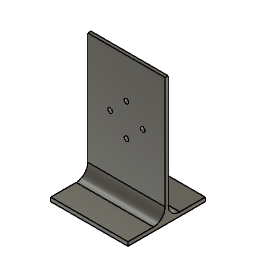
support-motor-v4 (Autodesk Fusion 360 design; units mm, degrees)
Autodesk Fusion 360 part; units mm, degrees
note: some values were not read from the file. Set by a fixed rule: which sketch regions a step uses.
sketch "Sketch1" plane through (0, 0, 0) normal (0, 0, 1) x (1, 0, 0)
  line L0 (0, 0) -> (50, 0)
  line L1 (50, 0) -> (50, 50)
  line L2 (50, 50) -> (0, 50)
  line L3 (0, 50) -> (0, 0)
  dimension "d3" = 50
  dimension "d4" = 50
  constraint horizontal L0
  constraint vertical L1
  constraint horizontal L2
  constraint vertical L3
  constraint coincident L0.start L3.end
  measures "d3" distance of L1.end L2.end
  measures "d4" distance of L0.start L2.end
extrude "Extrude1" add sketch "Sketch1" along normal blind 2.5
sketch "Sketch2" plane through (0, 0, 2.5) normal (0, 0, 1) x (-1, 0, 0)
  line L0 (0, -50) -> (0, 0)
  line L1 (0, 0) -> (-50, 0)
  line L2 (-50, 0) -> (-50, -50)
  line L3 (-50, -50) -> (0, -50)
  line L4 (0, -25) -> (-50, -25)
  line L5 (0, -26) -> (-50, -26)
  line L6 (-50, -26) -> (-50, -24)
  line L7 (-50, -24) -> (0, -24)
  line L8 (0, -24) -> (0, -26)
  dimension "d5" = 1
  dimension "d6" = 1
  constraint midpoint L0 L4.start
  constraint midpoint L2 L4.end
  constraint horizontal L5
  constraint vertical L6
  constraint horizontal L7
  constraint vertical L8
  constraint coincident L2 L6.end
  constraint coincident L0 L5.start
  measures "d5" distance of L4 L5
  measures "d6" distance of L4 L7
extrude "Extrude2" add sketch "Sketch2" along normal blind 80 contours L0 L2 L4 L5 L6 L8 | L0 L2 L4 L6 L7 L8
fillet "Fillet1" radius 7.5 2 edges at (25, 24, 2.5) (25, 26, 2.5)
sketch "Sketch3" plane through (0, 24, 0) normal (0, -1, 0) x (1, 0, 0)
  line L0 (0, 10) -> (50, 10)
  line L1 (50, 10) -> (50, 82.5)
  line L2 (50, 82.5) -> (0, 82.5)
  line L3 (0, 82.5) -> (0, 10)
  line L4 (0, 46.25) -> (50, 46.25)
  line L5 (25, 82.5) -> (25, 0)
  circle A0 centre (25, 56.75) radius 1.5
  circle A1 centre (14.5, 46.25) radius 1.5
  circle A2 centre (35.5, 46.25) radius 1.5
  circle A3 centre (25, 35.75) radius 1.5
  dimension "d11" = 3
  dimension "d12" = 10.5
  dimension "d13" = 3
  dimension "d14" = 10.5
  constraint midpoint L3 L4.start
  constraint midpoint L1 L4.end
  constraint midpoint L2 L5.start
  constraint perpendicular L2 L5
  constraint coincident L5 A0.centre
  constraint coincident L4 A1.centre
  constraint symmetric L5 A1 A2
  constraint symmetric L4 A0 A3
  measures "d11" diameter of A0
  measures "d12" distance of L4 A0.centre
  measures "d13" diameter of A1
  measures "d14" distance of L5 A1.centre
extrude "Extrude3" cut sketch "Sketch3" against normal blind 3 contours L5 A3 | L5 A3 | L4 A1 | L4 A1 | L4 A2 | L4 A2 | L5 A0 | L5 A0
